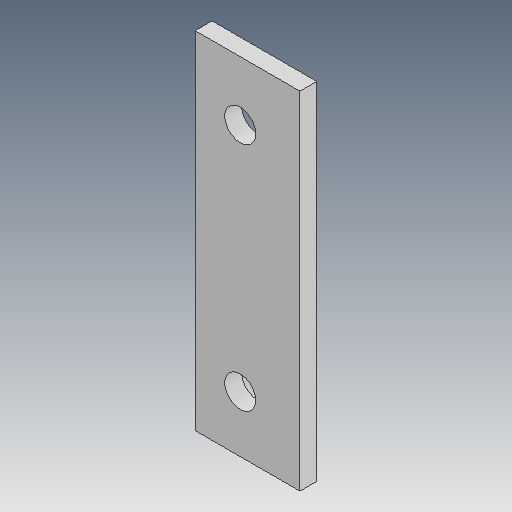
# Autodesk Inventor part: pulley_tab_left_B
Saved by Autodesk Inventor 2025.2 (Build 292293000, 293)
## iProperties
Created: 2025-02-16
Part Number: pulley_tab_left_B
Material: Generic
Document SubType Name: Modeling
Designer: email
Density: 1 g/cm^3
Appearance: Default
Author: email
Autodesk Inventor part; units mm, degrees
ref_plane "YZ Plane" through (0, 0, 0) normal (1, 0, 0) x (0, 1, 0)
ref_plane "XZ Plane" through (0, 0, 0) normal (0, 1, 0) x (-1, 0, 0)
ref_plane "XY Plane" through (0, 0, 0) normal (0, 0, 1) x (1, 0, 0)
sketch "Sketch1" plane through (0, 0, 0) normal (0, 0, 1) x (1, 0, 0)
  line L0 (0, 0) -> (18.6, 0)
  line L1 (18.6, 0) -> (18.6, 61.5)
  line L2 (18.6, 61.5) -> (0, 61.5)
  line L3 (0, 61.5) -> (0, 0)
  circle A0 centre (8, 10) radius 2.7436
  circle A1 centre (8, 51) radius 2.7436
  dimension "d0" = 61.5
  dimension "d1" = 18.6
  dimension "d2" = 10
  dimension "d3" = 8
  dimension "d4" = 8
  dimension "d5" = 10.5
  constraints: 8 end point, 2 centre point, 2 parallel, 1 equal radius, 1 horizontal, 1 perpendicular
  measures "d0" distance of L0.end L1.end
  measures "d1" distance of L1.end L2.end
  measures "d2" distance from line of L0 A0.centre
  measures "d3" distance from line of L3 A0.centre
  measures "d4" distance from line of L3 A1.centre
  measures "d5" distance from line of L2 A1.centre
extrude "Extrusion1" add sketch "Sketch1" along normal blind 3
body "Solid1"
